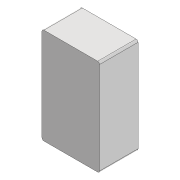
# Autodesk Inventor part: motor_dc_12v_90d
Saved by Autodesk Inventor 2020.2 (Build 242310000, 310)
## iProperties
Created: 2020-04-13
Part Number: motor_dc_12v_90d
Material: Generic
Document SubType Name: Modeling
Designer: Bardo91
Density: 1 g/cm^3
Appearance: Default
Author: Bardo91
Autodesk Inventor part; units mm, degrees
ref_plane "YZ Plane" through (0, 0, 0) normal (1, 0, 0) x (0, 1, 0)
ref_plane "XZ Plane" through (0, 0, 0) normal (0, 1, 0) x (-1, 0, 0)
ref_plane "XY Plane" through (0, 0, 0) normal (0, 0, 1) x (1, 0, 0)
sketch "Sketch1" plane through (0, 0, 0) normal (0, 0, 1) x (1, 0, 0)
  line L0 (0, 0) -> (14, 0)
  line L1 (15, 1) -> (15, 49)
  line L2 (14, 50) -> (-14, 50)
  line L3 (-15, 49) -> (-15, 1)
  line L4 (-14, 0) -> (15, 0)
  arc A0 (-14, 50) -> (-15, 49) centre (-14, 49) ccw
  arc A1 (15, 49) -> (14, 50) centre (14, 49) ccw
  arc A2 (14, 0) -> (15, 1) centre (14, 1) ccw
  arc A3 (-15, 1) -> (-14, 0) centre (-14, 1) ccw
  point P0 (15, 50)
  point P1 (-15, 50)
  dimension "d0" = 15
  dimension "d1" = 50
  dimension "d2" = 30
  dimension "d3" = 1
  constraints: 10 end point, 8 point on circle, 8 tangent, 6 point on line, 4 centre point, 3 equal radius, 2 horizontal, 1 collinear, 1 perpendicular, 1 vertical
  measures "d0" distance of L0.start L4.end
  measures "d1" distance of L4.end point (15, 50)
  measures "d2" distance of point (15, 50) point (-15, 50)
  measures "d3" radius of A0
extrude "Extrusion1" add sketch "Sketch1" along normal blind 20
body "Solid1"
